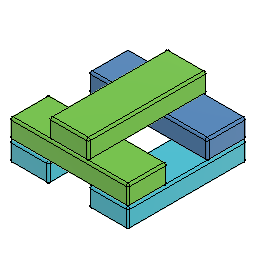
09-LinkedComponentsComplex (Autodesk Fusion 360 archive; units mm, degrees)
design "09-LinkedComponentsComplex-Data"
Autodesk Fusion 360 part; units mm, degrees
sketch "Sketch1" plane through (0, 0, 0) normal (0, 0, 1) x (1, 0, 0)
  line L0 (-30, 10) -> (30, 10)
  line L1 (30, 10) -> (30, 30)
  line L2 (30, 30) -> (-30, 30)
  line L3 (-30, 30) -> (-30, 10)
  line L4 (-30, 10) -> (30, 30) construction
  line L5 (30, 10) -> (-30, 30) construction
  point P0 (30, 10)
  point P1 (0, 20)
  dimension "d14" = 20
  dimension "d15" = 60
  constraint horizontal L0
  constraint perpendicular L0 L1
  constraint parallel L0 L2
  constraint parallel L1 L3
  constraint coincident L4 P1
  constraint coincident L5 P1
  constraint coincident P0 L0.end
  measures "d14" distance of P0 L1.end
  measures "d15" distance of L1.end L2.end
extrude "Extrude1" add sketch "Sketch1" along normal blind 10 makes body 1
sketch "Sketch1 (2)" plane through (0, 0, 0) normal (0, 0, 1) x (1, 0, 0) in component "mixed"
  line L0 (-30, 10) -> (30, 10)
  line L1 (30, 10) -> (30, 30)
  line L2 (30, 30) -> (-30, 30)
  line L3 (-30, 30) -> (-30, 10)
  line L4 (-30, 10) -> (30, 30) construction
  line L5 (30, 10) -> (-30, 30) construction
  point P0 (30, 10)
  point P1 (0, 20)
  dimension "d14_2" = 20
  dimension "d15_2" = 60
  constraint horizontal L0
  constraint perpendicular L0 L1
  constraint parallel L0 L2
  constraint parallel L1 L3
  constraint coincident L4 P1
  constraint coincident L5 P1
  constraint coincident P0 L0.end
  measures "d14_2" distance of P0 L1.end
  measures "d15_2" distance of L1.end L2.end
extrude "Extrude1'" add sketch "Sketch1 (2)" along normal blind 10 separate body makes body 2 in component "mixed"
sketch "Sketch1 (3)" plane through (0, 0, 0) normal (0, 0, 1) x (1, 0, 0) in component "subComponentWithBodies"
  line L0 (-30, 10) -> (30, 10)
  line L1 (30, 10) -> (30, 30)
  line L2 (30, 30) -> (-30, 30)
  line L3 (-30, 30) -> (-30, 10)
  line L4 (-30, 10) -> (30, 30) construction
  line L5 (30, 10) -> (-30, 30) construction
  point P0 (30, 10)
  point P1 (0, 20)
  dimension "d14_3" = 20
  dimension "d15_3" = 60
  constraint horizontal L0
  constraint perpendicular L0 L1
  constraint parallel L0 L2
  constraint parallel L1 L3
  constraint coincident L4 P1
  constraint coincident L5 P1
  constraint coincident P0 L0.end
  measures "d14_3" distance of P0 L1.end
  measures "d15_3" distance of L1.end L2.end
extrude "Extrude1''" add sketch "Sketch1 (3)" along normal blind 10 separate body makes body 3 in component "subComponentWithBodies"
sketch "Sketch1 (4)" plane through (0, 0, 0) normal (0, 0, 1) x (1, 0, 0) in component "hiddenComponent"
  line L0 (-30, 10) -> (30, 10)
  line L1 (30, 10) -> (30, 30)
  line L2 (30, 30) -> (-30, 30)
  line L3 (-30, 30) -> (-30, 10)
  line L4 (-30, 10) -> (30, 30) construction
  line L5 (30, 10) -> (-30, 30) construction
  point P0 (30, 10)
  point P1 (0, 20)
  dimension "d14_4" = 20
  dimension "d15_4" = 60
  constraint horizontal L0
  constraint perpendicular L0 L1
  constraint parallel L0 L2
  constraint parallel L1 L3
  constraint coincident L4 P1
  constraint coincident L5 P1
  constraint coincident P0 L0.end
  measures "d14_4" distance of P0 L1.end
  measures "d15_4" distance of L1.end L2.end
extrude "Extrude1'''" add sketch "Sketch1 (4)" along normal blind 10 separate body makes body 4 in component "hiddenComponent"
sketch "Sketch1 (5)" plane through (0, 0, 0) normal (0, 0, 1) x (1, 0, 0) in component "hiddenBodyFolder"
  line L0 (-30, 10) -> (30, 10)
  line L1 (30, 10) -> (30, 30)
  line L2 (30, 30) -> (-30, 30)
  line L3 (-30, 30) -> (-30, 10)
  line L4 (-30, 10) -> (30, 30) construction
  line L5 (30, 10) -> (-30, 30) construction
  point P0 (30, 10)
  point P1 (0, 20)
  dimension "d14_5" = 20
  dimension "d15_5" = 60
  constraint horizontal L0
  constraint perpendicular L0 L1
  constraint parallel L0 L2
  constraint parallel L1 L3
  constraint coincident L4 P1
  constraint coincident L5 P1
  constraint coincident P0 L0.end
  measures "d14_5" distance of P0 L1.end
  measures "d15_5" distance of L1.end L2.end
extrude "Extrude1''''" add sketch "Sketch1 (5)" along normal blind 10 separate body makes body 5 in component "hiddenBodyFolder"
sketch "Sketch1 (6)" plane through (0, 0, 0) normal (0, 0, 1) x (1, 0, 0) in component "hiddenBody"
  line L0 (-30, 10) -> (30, 10)
  line L1 (30, 10) -> (30, 30)
  line L2 (30, 30) -> (-30, 30)
  line L3 (-30, 30) -> (-30, 10)
  line L4 (-30, 10) -> (30, 30) construction
  line L5 (30, 10) -> (-30, 30) construction
  point P0 (30, 10)
  point P1 (0, 20)
  dimension "d14_6" = 20
  dimension "d15_6" = 60
  constraint horizontal L0
  constraint perpendicular L0 L1
  constraint parallel L0 L2
  constraint parallel L1 L3
  constraint coincident L4 P1
  constraint coincident L5 P1
  constraint coincident P0 L0.end
  measures "d14_6" distance of P0 L1.end
  measures "d15_6" distance of L1.end L2.end
extrude "Extrude1'''''" add sketch "Sketch1 (6)" along normal blind 10 separate body makes body 6 in component "hiddenBody"
copy_body "CopyPasteBodies1" bodies 3 makes body 7 in component "subComponentWithBodies"
move_body "Move1" bodies 7 to x (0, 1, 0) y (-1, 0, 0) z (0, 0, 1) at (20, 40, 10) in component "subComponentWithBodies"
fillet "Fillet1" radius 1 4 faces at (-10, 10, 3.3333) (-10, 23.3333, 10) (10, 30, 3.3333) (-10, 23.3333, 0) on bodies 1
fillet "Fillet1'" radius 1 8 faces at (-10, 23.3333, 10) (10, 30, 3.3333) (-10, 10, 3.3333) (-10, 23.3333, 0) (3.3333, 30, 20) (10, 30, 13.3333) (-10, 50, 13.3333) (3.3333, 30, 10) on bodies 3 7 in component "subComponentWithBodies"
fillet "Fillet1''" radius 1 4 faces at (-10, 23.3333, 10) (-10, 23.3333, 0) (10, 30, 3.3333) (-10, 10, 3.3333) on bodies 2 in component "mixed"
component "deep" placed x (1, 0, 0) y (0, 1, 0) z (0, 0, 1) at (0, 0, 0) in component "09-LinkedComponentsComplex v0"
component "renamedBlock" placed x (1, 0, 0) y (0, 1, 0) z (0, 0, 1) at (0, 0, 0) in component "09-LinkedComponentsComplex v0"
component "mixed" placed x (1, 0, 0) y (0, 1, 0) z (0, 0, 1) at (0, 0, 0) in component "09-LinkedComponentsComplex v0"
component "hiddenComponent" placed x (1, 0, 0) y (0, 1, 0) z (0, 0, 1) at (0, 0, 0) in component "09-LinkedComponentsComplex v0"
component "hiddenBodyFolder" placed x (1, 0, 0) y (0, 1, 0) z (0, 0, 1) at (0, 0, 0) in component "09-LinkedComponentsComplex v0"
component "hiddenBody" placed x (1, 0, 0) y (0, 1, 0) z (0, 0, 1) at (0, 0, 0) in component "09-LinkedComponentsComplex v0"
component "deeper" placed x (1, 0, 0) y (0, 1, 0) z (0, 0, 1) at (0, 0, 0) in component "deep"
component "deepest" placed x (1, 0, 0) y (0, 1, 0) z (0, 0, 1) at (0, 0, 0) in component "deeper"
component "renamedBlock" placed x (1, 0, 0) y (0, 1, 0) z (0, 0, 1) at (0, 0, 0) in component "deepest"
component "subComponentWithBodies" placed x (1, 0, 0) y (0, 1, 0) z (0, 0, 1) at (0, 0, 0) in component "mixed"
hidden bodies 6
named bodies: "bodyInComponentWithSubComponents", "hiddenComponent", "hiddenBodyFolder", "hiddenBody"
